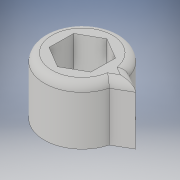
# Autodesk Inventor part: toggle
Saved by Autodesk Inventor 2018.1 (Build 221171000, 171)
## iProperties
Created: 2017-11-21
Part Number: toggle
Material: Generic
Document SubType Name: Modeling
Designer: bramd
Density: 1 g/cm^3
Appearance: Default
Author: bramd
Autodesk Inventor part; units mm, degrees
ref_plane "YZ Plane" through (0, 0, 0) normal (1, 0, 0) x (0, 1, 0)
ref_plane "XZ Plane" through (0, 0, 0) normal (0, 1, 0) x (-1, 0, 0)
ref_plane "XY Plane" through (0, 0, 0) normal (0, 0, 1) x (1, 0, 0)
sketch "Sketch1" plane through (0, 0, 0) normal (0, 1, 0) x (-1, 0, 0)
  circle A0 centre (0, 0) radius 5
  dimension "d0" = 10
  constraints: 1 centre point, 1 coincident
  measures "d0" diameter of A0
sketch "Sketch2" plane through (0, 0, 0) normal (0, 1, 0) x (-1, 0, 0)
  line L0 (2.7746, -1.6463) -> (-0.0384, -3.226)
  line L1 (-0.0384, -3.226) -> (-2.813, -1.5797)
  line L2 (-2.813, -1.5797) -> (-2.7746, 1.6463)
  line L3 (-2.7746, 1.6463) -> (0.0384, 3.226)
  line L4 (0.0384, 3.226) -> (2.813, 1.5797)
  line L5 (2.813, 1.5797) -> (2.7746, -1.6463)
  point P0 (0, 0)
  dimension "d5" = 5.588
  constraints: 12 end point, 13 other
  measures "d5" distance between parallel lines of L2 L5
sketch "Sketch3" plane through (0, 0, 0) normal (0, 1, 0) x (-1, 0, 0)
  point P0 (0, 0)
extrude "Extrusion1" add sketch "Sketch1" along normal blind 7.5
extrude "Extrusion2" cut sketch "Sketch2" along normal blind 7.5
sketch "Sketch4" plane through (0, 7.5, 0) normal (0, 1, 0) x (1, 0, 0)
  circle A0 centre (0, 0) radius 5 projected
  line L0 (7.0477, 0) -> (3.9762, -1.7733)
  line L1 (3.9762, -1.7733) -> (3.9762, 1.7733)
  line L2 (3.9762, 1.7733) -> (7.0477, 0)
  point P0 (5, 0)
  constraints: 6 end point, 1 horizontal alignment, 8 other
extrude "Extrusion3" add sketch "Sketch4" against normal blind 7.5 contours A0 L0 L1 L2 | A0 L2 L0 picked at (4.3175, 0)
fillet "Fillet1" radius 1 1 edges at (-5, 7.5, 0)
fillet "Fillet2" radius 1 4 edges at (4.1175, 7.5, 1.6917) (5.9408, 7.5, 0.6391) (4.1175, 7.5, -1.6917) (5.9408, 7.5, -0.6391)
body "Solid1"
